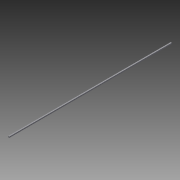
# Autodesk Inventor part: Lower Goal Longer
Saved by Autodesk Inventor 2014 (Build 180170000, 170)
## iProperties
Created: 2014-01-29
Part Number: Lower Goal Longer
Material: Generic
Document SubType Name: Modeling
Designer: NilesStanton
Density: 1 g/cm^3
Appearance: Default
Author: NilesStanton
Autodesk Inventor part; units mm, degrees
ref_plane "YZ Plane" through (0, 0, 0) normal (1, 0, 0) x (0, 1, 0)
ref_plane "XZ Plane" through (0, 0, 0) normal (0, 1, 0) x (-1, 0, 0)
ref_plane "XY Plane" through (0, 0, 0) normal (0, 0, 1) x (1, 0, 0)
sketch "Sketch1" plane through (0, 0, 0) normal (0, 1, 0) x (-1, 0, 0)
  line L0 (-13.6663, 926.6859) -> (-7.3163, 926.6859)
  line L1 (-7.3163, 926.6859) -> (-7.3163, -6.7641)
  line L2 (-7.3163, -6.7641) -> (-13.6663, -6.7641)
  line L3 (-13.6663, -6.7641) -> (-13.6663, 926.6859)
  point P0 (0, 0)
  dimension "d0" = 6.35
  dimension "d1" = 933.45
  constraints: 8 end point, 2 parallel, 1 horizontal, 1 perpendicular
  measures "d0" distance of L1.end L2.end
  measures "d1" distance of L0.end L1.end
extrude "Extrusion1" add sketch "Sketch1" along normal blind 6.35
body "Solid1"
